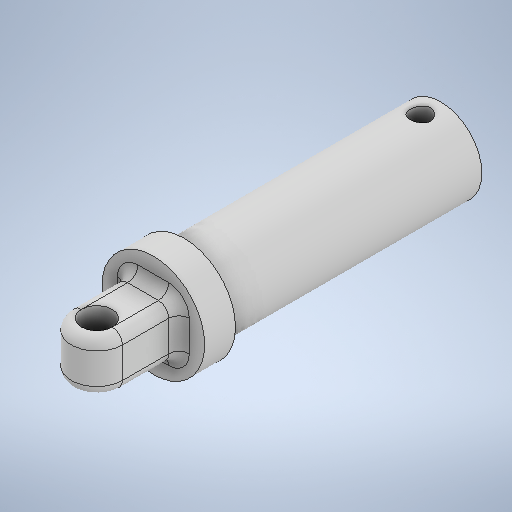
# Autodesk Inventor part: SuspensionCap
Saved by Autodesk Inventor 2025.2 (Build 292293000, 293)
## iProperties
Created: 2025-01-06
Part Number: SuspensionCap
Material: 일반
Document SubType Name: Modeling
Designer: SEON
Density: 1 g/cm^3
Appearance: 기본값
Author: SEON
Autodesk Inventor part; units mm, degrees
ref_plane "YZ Plane" through (0, 0, 0) normal (1, 0, 0) x (0, 1, 0)
ref_plane "XY Plane" through (0, 0, 0) normal (0, 0, 1) x (1, 0, 0)
sketch "스케치1" plane through (0, 0, 0) normal (0, 0, 1) x (1, 0, 0)
  circle A0 centre (0, 0) radius 5
  dimension "d0" = 10
  constraints: 1 centre point, 1 coincident
  measures "d0" diameter of A0
extrude "돌출1" add sketch "스케치1" along normal blind 3
ref_plane "작업 평면1" through (0, 0, 0) normal (0, 1, 0) x (-1, 0, 0)
sketch "스케치2" plane through (0, 0, 0) normal (0, 1, 0) x (-1, 0, 0)
  line L0 (5, 3) -> (-5, 3) projected
  line L1 (2.5, 3) -> (-2.5, 3)
  line L2 (-2.5, 3) -> (-2.5, 11)
  line L3 (-2.5, 11) -> (2.5, 11)
  line L4 (2.5, 11) -> (2.5, 3)
  circle A0 centre (0, 8.5) radius 1.5
  point P0 (0, 0)
  point P1 (0, 3)
  point P2 (0, 11)
  dimension "d3" = 5
  dimension "d4" = 8
  dimension "d5" = 3
  dimension "d19" = 2.5
  constraints: 8 end point, 2 midpoint, 2 parallel, 2 vertical alignment, 1 centre point, 1 horizontal, 1 perpendicular, 1 point on line
  measures "d3" distance of L2.end L3.end
  measures "d4" distance of L3.end L1.start
  measures "d5" diameter of A0
  measures "d19" distance of A0.centre point (0, 11)
extrude "돌출2" add sketch "스케치2" along normal mid plane 5
fillet "모깎기1" radius 2.5 2 edges at (2.5, 0, 11) (-2.5, 0, 11)
fillet "모깎기2" radius 1 10 edges at (0, 2.5, 11) (-1.7678, 2.5, 10.2678) (1.7678, 2.5, 10.2678) (2.5, 2.5, 5.75) (-2.5, 2.5, 5.75) (-1.7678, -2.5, 10.2678) (0, -2.5, 11) (1.7678, -2.5, 10.2678) (2.5, -2.5, 5.75) (-2.5, -2.5, 5.75)
fillet "모깎기3" radius 1 8 edges at (-2.2071, -2.2071, 3) (-2.5, 0, 3) (-2.2071, 2.2071, 3) (0, 2.5, 3) (2.2071, 2.2071, 3) (2.5, 0, 3) (2.2071, -2.2071, 3) (0, -2.5, 3)
sketch "스케치3" plane through (0, 0, 0) normal (0, 0, -1) x (-1, 0, 0)
  circle A0 centre (0, 0) radius 4
  circle A1 centre (0, 0) radius 2.5
  dimension "d11" = 8
  dimension "d12" = 5
  constraints: 2 centre point, 2 coincident
  measures "d11" diameter of A0
  measures "d12" diameter of A1
extrude "돌출3" add sketch "스케치3" along normal blind 25
ref_plane "작업 평면2" through (0, 4, 0) normal (0, 1, 0) x (-1, 0, 0)
sketch "스케치4" plane through (0, 4, 0) normal (0, 1, 0) x (-1, 0, 0)
  circle A0 centre (0, -23) radius 1
  line L0 (-4, -25) -> (4, -25) projected
  point P0 (0, 0)
  dimension "d15" = 2
  dimension "d16" = 2
  constraints: 1 centre point, 1 vertical alignment
  measures "d15" diameter of A0
  measures "d16" distance from line of L0 A0.centre
extrude "돌출4" cut sketch "스케치4" against normal through all
